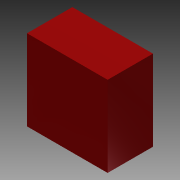
# Autodesk Inventor part: USB_Cap
Saved by Autodesk Inventor 2015 (Build 190159000, 159)
## iProperties
Created: 2013-02-26
Part Number: USB_Cap
Material: Generic
Document SubType Name: Modeling
Density: 1 g/cm^3
Appearance: Red
Autodesk Inventor part; units mm, degrees
ref_plane "YZ Plane" through (0, 0, 0) normal (1, 0, 0) x (0, 1, 0)
ref_plane "XZ Plane" through (0, 0, 0) normal (0, 1, 0) x (-1, 0, 0)
ref_plane "XY Plane" through (0, 0, 0) normal (0, 0, 1) x (1, 0, 0)
sketch "Sketch1" plane through (0, 0, 0) normal (0, 0, 1) x (1, 0, 0)
  line L0 (0, 11.2) -> (0, -11.2) projected
  line L1 (-11.2, 0) -> (11.2, 0) projected
  line L2 (-8, 8) -> (8, 8)
  line L3 (8, 8) -> (8, -8)
  line L4 (8, -8) -> (-8, -8)
  line L5 (-8, -8) -> (-8, 8)
  dimension "d0" = 16
  dimension "d1" = 16
  constraints: 8 end point, 2 parallel, 1 horizontal, 1 perpendicular, 2 other
  measures "d0" distance of L2.start L2.end
  measures "d1" distance of L4.end L2.start
extrude "BLOK" add sketch "Sketch1" along normal mid plane 9
sketch "Sketch3" plane through (-8, -8, 4.5) normal (-1, 0, 0) x (0, 0, 1)
  line L0 (0, 0) -> (-9, 0) projected
  line L1 (-9, 16) -> (0, 16) projected
  line L2 (-9, 0) -> (-9, 16) projected
  line L3 (-7, 15) -> (-2, 15)
  line L4 (-2, 15) -> (-2, 1)
  line L5 (-2, 1) -> (-7, 1)
  line L6 (-7, 1) -> (-7, 15)
  point P0 (-4.5, 8)
  dimension "d21" = 2
  dimension "d22" = 1
  dimension "d23" = 1
  dimension "d24" = 5
  constraints: 8 end point, 2 parallel, 1 horizontal, 1 perpendicular
  measures "d21" distance between parallel lines of L2 L6
  measures "d22" distance between parallel lines of L1 L3
  measures "d23" distance between parallel lines of L0 L5
  measures "d24" distance between parallel lines of L6 L4
extrude "USBGAT" cut sketch "Sketch3" against normal blind 12
body "Solid1"
